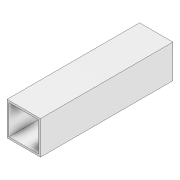
# Autodesk Inventor part: Pasabable Ranurado 30 x 30 L = 430
Saved by Autodesk Inventor 2020 (Build 240168000, 168)
## iProperties
Created: 2020-07-02
Part Number: Pasabable Ranurado 30 x 30 L = 430
Material: PVC-Piping
Document SubType Name: Modeling
Designer: Hernan
Density: 1.4 g/cm^3
Appearance: Smooth - White
Author: Hernan
Autodesk Inventor part; units mm, degrees
ref_plane "YZ Plane" through (0, 0, 0) normal (1, 0, 0) x (0, 1, 0)
ref_plane "XZ Plane" through (0, 0, 0) normal (0, 1, 0) x (-1, 0, 0)
ref_plane "XY Plane" through (0, 0, 0) normal (0, 0, 1) x (1, 0, 0)
sketch "Sketch1" plane through (0, 0, 0) normal (0, 0, 1) x (1, 0, 0)
  line L0 (-26.9918, -9.5406) -> (3.0082, -9.5406)
  line L1 (3.0082, -9.5406) -> (3.0082, 20.4594)
  line L2 (3.0082, 20.4594) -> (-26.9918, 20.4594)
  line L3 (-26.9918, 20.4594) -> (-26.9918, -9.5406)
  line L4 (1.3082, 20.4594) -> (1.3082, -9.5406)
  line L5 (-26.9918, -7.8406) -> (3.0082, -7.8406)
  line L6 (-25.2918, 20.4594) -> (-25.2918, -9.5406)
  line L7 (-26.9918, 18.7594) -> (3.0082, 18.7594)
  point P0 (0, 0)
  point P1 (1.3082, 18.7594)
  point P2 (-25.2918, 18.7594)
  point P3 (-25.2918, -7.8406)
  point P4 (1.3082, -7.8406)
  dimension "d0" = 30
  dimension "d1" = 30
  dimension "d4" = 1.7
  dimension "d5" = 1.7
  dimension "d6" = 1.7
  dimension "d7" = 1.7
  constraints: 16 end point, 8 point on line, 3 horizontal, 3 perpendicular, 2 vertical
  measures "d0" distance of L0.start L0.end
  measures "d1" distance of L0.end L1.end
  measures "d4" distance between parallel lines of L2 L7
  measures "d5" distance between parallel lines of L3 L6
  measures "d6" distance between parallel lines of L0 L5
  measures "d7" distance between parallel lines of L1 L4
extrude "Extrusion1" add sketch "Sketch1" against normal blind 119.059
extrude "Extrusion2" cut sketch "Sketch1" against normal blind 160 contours L6 L7 L4 L5
body "Solid1"
